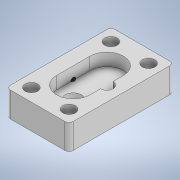
# Autodesk Inventor part: Część6
Saved by Autodesk Inventor 2021 (Build 250183000, 183)
## iProperties
Created: 2023-09-22
Part Number: Część6
Material: Ogólny
Document SubType Name: Modeling
Designer: Jakub
Density: 1 g/cm^3
Appearance: Domyślna
Author: Jakub
Autodesk Inventor part; units mm, degrees
ref_plane "YZ Plane" through (0, 0, 0) normal (1, 0, 0) x (0, 1, 0)
ref_plane "XZ Plane" through (0, 0, 0) normal (0, 1, 0) x (-1, 0, 0)
ref_plane "XY Plane" through (0, 0, 0) normal (0, 0, 1) x (1, 0, 0)
sketch "Szkic1" plane through (0, 0, 0) normal (0, 1, 0) x (-1, 0, 0)
  line L0 (0, 0) -> (-15, 0)
  line L1 (-15, 0) -> (-15, -25)
  line L2 (-15, -25) -> (0, -25)
  line L3 (0, -25) -> (0, 0)
  dimension "d0" = 15
  dimension "d1" = 25
  constraints: 8 end point, 3 perpendicular, 1 horizontal
  measures "d0" distance of L0.start L0.end
  measures "d1" distance of L0.end L1.end
extrude "Wyciągnięcie proste1" add sketch "Szkic1" along normal blind 3
sketch "Szkic2" plane through (0, 3, 0) normal (0, 1, 0) x (1, 0, 0)
  line L0 (0, 25) -> (0, 0) projected
  line L1 (0, 0) -> (15, 0) projected
  line L2 (0, 0) -> (15, 0)
  line L3 (15, 0) -> (15, 25) projected
  line L4 (15, 0) -> (15, 25)
  line L5 (15, 25) -> (0, 25)
  line L6 (0, 25) -> (0, 0)
  line L7 (3.5, 4.5) -> (3.5, 20.5)
  line L8 (3.5, 20.5) -> (11.5, 20.5)
  line L9 (11.5, 20.5) -> (11.5, 4.5)
  line L10 (11.5, 4.5) -> (3.5, 4.5)
  dimension "d4" = 16
  dimension "d5" = 8
  dimension "d6" = 16
  constraints: 16 end point, 4 perpendicular, 2 collinear, 1 vertical
  measures "d4" distance of L7.start L7.end
  measures "d5" distance of L7.end L8.end
  measures "d6" distance of L8.end L9.end
extrude "Wyciągnięcie proste2" add sketch "Szkic2" along normal blind 3
fillet "Zaokrąglenie1" radius 4 1 edges at (11.5, 4.5, -20.5)
fillet "Zaokrąglenie2" radius 4 1 edges at (3.5, 4.5, -20.5)
fillet "Zaokrąglenie3" radius 4 1 edges at (3.5, 4.5, -4.5)
fillet "Zaokrąglenie4" radius 4 1 edges at (11.5, 4.5, -4.5)
fillet "Zaokrąglenie5" radius 1 1 edges at (15, 3, -25)
fillet "Zaokrąglenie6" radius 1 1 edges at (0, 3, -25)
fillet "Zaokrąglenie7" radius 1 1 edges at (0, 3, 0)
fillet "Zaokrąglenie8" radius 1 1 edges at (15, 3, 0)
sketch "Szkic3" plane through (0, 6, 0) normal (0, 1, 0) x (1, 0, 0)
  line L0 (3, 3) -> (3, 22)
  line L1 (3, 22) -> (12, 22)
  line L2 (12, 22) -> (12, 3)
  line L3 (12, 3) -> (3, 3)
  circle A0 centre (3, 3) radius 1.5
  circle A1 centre (12, 3) radius 1.5
  circle A2 centre (12, 22) radius 1.5
  circle A3 centre (3, 22) radius 1.5
  point P0 (0, 0)
  dimension "d17" = 19
  dimension "d18" = 9
  dimension "d19" = 19
  dimension "d20" = 3
  dimension "d21" = 3
  dimension "d22" = 3
  dimension "d23" = 3
  constraints: 8 end point, 4 centre point, 4 coincident, 2 perpendicular, 1 vertical
  measures "d17" distance of L0.start L0.end
  measures "d18" distance of L0.end L1.end
  measures "d19" distance of L1.end L2.end
  measures "d20" diameter of A0
  measures "d21" diameter of A1
  measures "d22" diameter of A2
  measures "d23" diameter of A3
extrude "Wyciągnięcie proste3" cut sketch "Szkic3" against normal blind 6 contours L3 A0 L0 | L0 A0 L3 | A3 L1 L0 | L0 L1 A3 | A1 L2 L3 | L3 L2 A1 | A2 L2 L1 | L1 L2 A2
sketch "Szkic6" plane through (0, 0, 0) normal (0, -1, 0) x (1, 0, 0)
  circle A0 centre (11.5, -12.5) radius 2.5
  point P0 (0, 0)
  dimension "d27" = 5
  constraints: 1 centre point
  measures "d27" diameter of A0
extrude "Wyciągnięcie proste4" cut sketch "Szkic6" against normal blind 3
sketch "Szkic7" plane through (0, 6, 0) normal (0, 1, 0) x (1, 0, 0)
  line L0 (11.5, 16.5) -> (11.5, 8.5) projected
  circle A0 centre (11.5, 12.5) radius 1.5
  point P0 (0, 0)
  point P1 (11.5, 14)
  point P2 (11.5, 11)
  dimension "d30" = 3
  constraints: 1 centre point, 1 midpoint
  measures "d30" diameter of A0
extrude "Wyciągnięcie proste5" cut sketch "Szkic7" against normal blind 3 contours A0 L0 picked at (11.9875, 12.6113)
sketch "Szkic8" plane through (0, 0, 0) normal (0, -1, 0) x (1, 0, 0)
  circle A0 centre (7.5, -8.5) radius 2
  point P0 (0, 0)
  dimension "d33" = 4
  constraints: 1 centre point
  measures "d33" diameter of A0
extrude "Wyciągnięcie proste6" cut sketch "Szkic8" against normal blind 3
sketch "Szkic11" plane through (0, 0, -24) normal (-1, 0, 0) x (0, 0, 1)
  line L0 (24, 6) -> (24, 0) projected
  line L1 (24, 3) -> (-1, 3)
  line L2 (-1, 6) -> (-1, 0) projected
  line L3 (7.5, 3) -> (15.5, 3) projected
  line L4 (11.5, 3) -> (11.5, 6)
  line L5 (10, 6) -> (13, 6) projected
  line L6 (11.5, 3) -> (11.5, 0)
  constraints: 6 end point, 4 midpoint, 1 point on line
hole "Otwór1" at (0, 3, -12.5) direction (1, 0, 0) diameter 3 depth 3 tip angle 120
sketch "Szkic13" plane through (0, 0, -24) normal (-1, 0, 0) x (0, 0, 1)
  line L0 (9, 3) -> (14, 3) projected
  circle A0 centre (11.5, 3) radius 2.5
  line L1 (14, 0) -> (14, 3) projected
  point P0 (24, 0)
  constraints: 1 centre point, 1 midpoint, 1 tangent
extrude "Wyciągnięcie proste7" cut sketch "Szkic13" against normal blind 1.5
